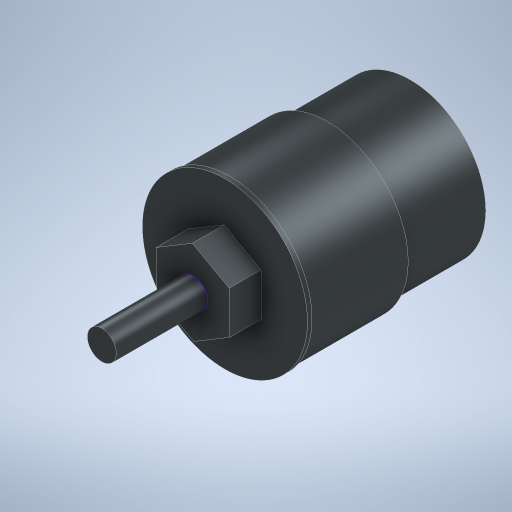
# Autodesk Inventor part: DC MOTOR1
Saved by Autodesk Inventor 2023 (Build 270158000, 158)
## iProperties
Created: 2022-06-10
Part Number: DC MOTOR1
Material: Iron, Gray
Document SubType Name: Modeling
Designer: TRIVENI MAGADUM
Density: 7.15 g/cm^3
Appearance: Iron Gray
Author: TRIVENI MAGADUM
Autodesk Inventor part; units mm, degrees
ref_plane "YZ Plane" through (0, 0, 0) normal (1, 0, 0) x (0, 1, 0)
ref_plane "XZ Plane" through (0, 0, 0) normal (0, 1, 0) x (-1, 0, 0)
ref_plane "XY Plane" through (0, 0, 0) normal (0, 0, 1) x (1, 0, 0)
sketch "Sketch1" plane through (0, 0, 0) normal (0, 0, 1) x (1, 0, 0)
  circle A0 centre (0, 0) radius 17.7488
  constraints: 1 centre point, 1 coincident
extrude "Extrusion1" add sketch "Sketch1" along normal blind 21.45
sketch "Sketch2" plane through (0, 0, 0) normal (0, 0, -1) x (-1, 0, 0)
  circle A0 centre (0, 0) radius 16.574
  constraints: 1 centre point, 1 coincident
extrude "Extrusion2" add sketch "Sketch2" along normal blind 18.2
sketch "Sketch5" plane through (0, 0, 21.45) normal (0, 0, 1) x (1, 0, 0)
  circle A0 centre (0, 0) radius 18.1003
  constraints: 1 centre point, 1 coincident
extrude "Extrusion5" add sketch "Sketch5" along normal blind 1
sketch "Sketch3" plane through (0, 0, -18.2) normal (0, 0, -1) x (-1, 0, 0)
  circle A0 centre (0, 0) radius 17.7488 projected
  line L0 (17.7488, 0) -> (14.2875, 0)
  circle A1 centre (0, 0) radius 16.574 projected
  line L1 (15.3093, 6.35) -> (15.3093, -6.35)
  circle A2 centre (3.175, 7.9375) radius 1.5875
  constraints: 4 end point, 2 point on circle, 1 centre point, 1 horizontal alignment, 1 vertical, 1 other
extrude "Extrusion3" add sketch "Sketch3" against normal blind 10 contours A2
sketch "Sketch4" plane through (0, 0, -18.2) normal (0, 0, -1) x (-1, 0, 0)
  circle A0 centre (3.175, -4.7625) radius 1.5875
  point P0 (0, 0)
  constraints: 1 centre point
extrude "Extrusion4" cut sketch "Sketch4" against normal blind 10
sketch "Sketch6" plane through (0, 0, 22.45) normal (0, 0, 1) x (1, 0, 0)
  point P0 (0, 0)
sketch "Sketch7" plane through (0, 0, 22.45) normal (0, 0, 1) x (1, 0, 0)
  line L0 (7.9375, 4.7625) -> (8.0932, -4.4928)
  line L1 (8.0932, -4.4928) -> (0.1557, -9.2553)
  line L2 (0.1557, -9.2553) -> (-7.9375, -4.7625)
  line L3 (-7.9375, -4.7625) -> (-8.0932, 4.4928)
  line L4 (-8.0932, 4.4928) -> (-0.1557, 9.2553)
  line L5 (-0.1557, 9.2553) -> (7.9375, 4.7625)
  point P0 (0, 0)
  point P1 (0, 0)
  constraints: 12 end point, 13 other
sketch "Sketch8" plane through (0, 0, 22.45) normal (0, 0, 1) x (1, 0, 0)
  point P0 (0, 0)
extrude "Extrusion6" add sketch "Sketch7" along normal blind 7
sketch "Sketch9" plane through (0, 0, 29.45) normal (0, 0, 1) x (1, 0, 0)
  circle A0 centre (0, 0) radius 3.175
  constraints: 1 centre point, 1 coincident
extrude "Extrusion7" add sketch "Sketch9" along normal blind 20
body "Solid1"
